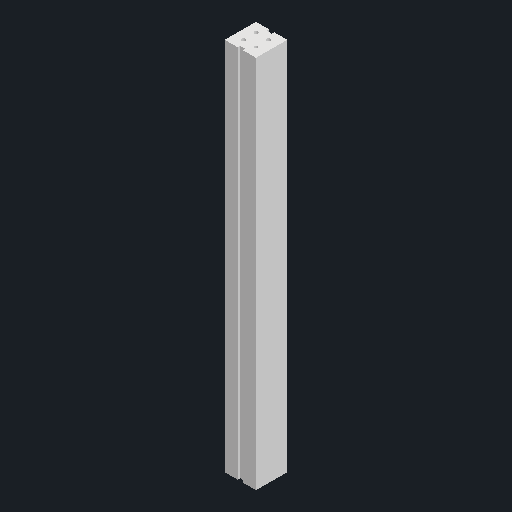
# Autodesk Inventor part: 1_inner_leg
Saved by Autodesk Inventor 2024 (Build 280153000, 153)
## iProperties
Created: 2023-05-22
Part Number: 1_inner_leg
Material: Generic
Document SubType Name: Modeling
Designer: aasmu
Density: 1 g/cm^3
Appearance: Default
d12: 600.000 mm
cabel_shaft_size: 4.000 mm
edge_to_hole: 15.000 mm
hole_diameter: 6.000 mm
inner_leg_width: 50.000 mm
height: 600.000 mm
Author: aasmu
Autodesk Inventor part; units mm, degrees
ref_plane "YZ Plane" through (0, 0, 0) normal (1, 0, 0) x (0, 1, 0)
ref_plane "XZ Plane" through (0, 0, 0) normal (0, 1, 0) x (-1, 0, 0)
ref_plane "XY Plane" through (0, 0, 0) normal (0, 0, 1) x (1, 0, 0)
sketch "Sketch3" plane through (0, 0, 0) normal (0, 1, 0) x (-1, 0, 0)
  line L0 (-56.572, -4.0671) -> (-56.572, -54.0671)
  line L1 (-6.572, -54.0671) -> (-6.572, -4.0671)
  line L2 (-6.572, -4.0671) -> (-35.572, -4.0671)
  line L3 (-35.572, -4.0671) -> (-35.572, -8.0671)
  line L4 (-35.572, -8.0671) -> (-27.572, -8.0671)
  line L5 (-27.572, -8.0671) -> (-27.572, -4.0671)
  line L6 (-27.572, -4.0671) -> (-56.572, -4.0671)
  line L7 (-6.572, -29.0671) -> (-22.7851, -29.0671) construction
  line L8 (-6.572, -54.0671) -> (-35.572, -54.0671)
  line L9 (-35.572, -54.0671) -> (-35.572, -50.0671)
  line L10 (-35.572, -50.0671) -> (-27.572, -50.0671)
  line L11 (-27.572, -50.0671) -> (-27.572, -54.0671)
  line L12 (-27.572, -54.0671) -> (-56.572, -54.0671)
  line L13 (-21.572, -4.0671) -> (-21.572, -19.0671) construction
  line L14 (-21.572, -19.0671) -> (-6.572, -19.0671) construction
  line L15 (-56.572, -19.0671) -> (-41.572, -19.0671) construction
  line L16 (-56.572, -39.0671) -> (-41.572, -39.0671) construction
  line L17 (-21.572, -54.0671) -> (-21.572, -39.0671) construction
  line L18 (-21.572, -39.0671) -> (-6.572, -39.0671) construction
  circle A0 centre (-21.572, -19.0671) radius 3
  circle A1 centre (-41.572, -19.0671) radius 3
  circle A2 centre (-41.572, -39.0671) radius 3
  circle A3 centre (-21.572, -39.0671) radius 3
  point P0 (-35.572, -4.0671)
  dimension "d36" = 50
  dimension "d37" = 50
  dimension "d38" = 4
  dimension "d40" = 15
  dimension "d41" = 6
  dimension "d46" = 8
  constraints: 38 end point, 9 point on line, 6 equal length, 6 perpendicular, 6 symmetric about line, 4 centre point, 4 coincident, 4 horizontal, 3 equal radius, 3 vertical, 2 collinear, 1 midpoint, 1 parallel, 1 other
  measures "d36" distance of L1.start L0.end
  measures "d37" distance of L0.end L0.start
  measures "d38" distance of L4.end L5.end
  measures "d40" distance of L13.start L13.end
  measures "d41" diameter of A0
  measures "d46" distance of L3.end L4.end
extrude "Extrusion3" add sketch "Sketch3" along normal blind 600 contours L6 L3 L4 L5 L2 L1 L8 L11 L10 L9 L12 L0 | A0 | A1 | A2 | A3
extrude "Extrusion6" cut sketch "Sketch3" along normal blind 30 contours A0 | A1 | A2 | A3
extrude "Extrusion7" cut sketch "Sketch3" against normal blind 30 from surface at 600 contours A0 | A1 | A2 | A3
equation "\"d36\" = inner_leg_width"
equation "\"d37\" = inner_leg_width"
equation "\"d38\" = cabel_shaft_size"
equation "\"d40\" = edge_to_hole"
equation "\"d41\" = hole_diameter"
equation "\"d46\" = 2 * cabel_shaft_size"
equation "\"d12\" = height"
equation "\"d42\" = hole_depth"
equation "\"d44\" = hole_depth"
equation "\"cabel_shaft_size\" = 4"
equation "\"edge_to_hole\" = 15"
equation "\"hole_diameter\" = 6"
equation "\"height\" = 600"
equation "\"inner_leg_width\" = 50"
equation "\"hole_depth\" = 30"
body "Solid2"
